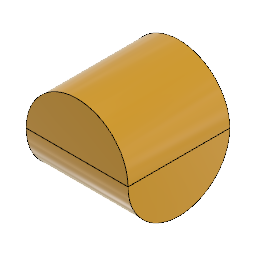
Dual Sphericon (Autodesk Fusion 360 design; units mm, degrees)
Autodesk Fusion 360 part; units mm, degrees
note: some values were not read from the file. Set by a fixed rule: which sketch regions a step uses.
sketch "Profile" plane through (0, 0, 0) normal (0, 0, 1) x (1, 0, 0)
  line L0 (50, 50) -> (-50, 50)
  line L1 (-50, 50) -> (-50, -50)
  line L2 (-50, -50) -> (50, -50)
  line L3 (50, -50) -> (50, 50)
  line L4 (-50, 0) -> (50, 0)
  dimension "d1" = 50
revolve "Revolve1" add sketch "Profile" angle 360 about axis through (-50, 0, 0) along (1, 0, 0) contours L0 L1 L3 L4 makes body 1
split "Split1" by plane through (0, 0, 0) normal (0, 0, 1) bodies 1 makes body 2 at (16.6667, -39.8566, 30.1902)
move_body "Move1" bodies 2 to x (0, -1, 0) y (1, 0, 0) z (0, 0, 1) at (0, 0, 0)
sketch "Holes" plane through (0, 0, 0) normal (0, 0, 1) x (1, 0, 0)
  circle A0 centre (0, 0) radius 5
  circle A1 centre (0, 0) radius 12.5
  circle A2 centre (12.5, 0) radius 2.6
  circle A3 centre (0, 12.5) radius 2.6
  circle A4 centre (-12.5, 0) radius 2.6
  circle A5 centre (0, -12.5) radius 2.6
  dimension "d4" = 10
  dimension "d5" = 25
  dimension "d6" = 5.2
  dimension "d8" = 360
  measures "d4" diameter of A0
  measures "d5" diameter of A1
  measures "d6" diameter of A2
extrude "Extrude1" cut sketch "Holes" along normal mid plane 32 contours A0 bodies 1 2
extrude "Extrude2" cut sketch "Holes" along normal mid plane 14 contours A1 A2 | A1 A2 | A1 A3 | A1 A3 | A1 A5 | A1 A5 | A1 A4 | A1 A4 bodies 1 2
chamfer "Chamfer1" distance 5 angle 45 1 edges at (-4.6616, -1.8081, 16) on bodies 2
chamfer "Chamfer2" distance 2.5 angle 45 4 edges at (-2.4241, -13.4402, 7) (10.0759, -0.9402, 7) (-2.4241, 11.5598, 7) (-14.9241, -0.9402, 7) on bodies 2
named bodies: "Bottom", "Top"
